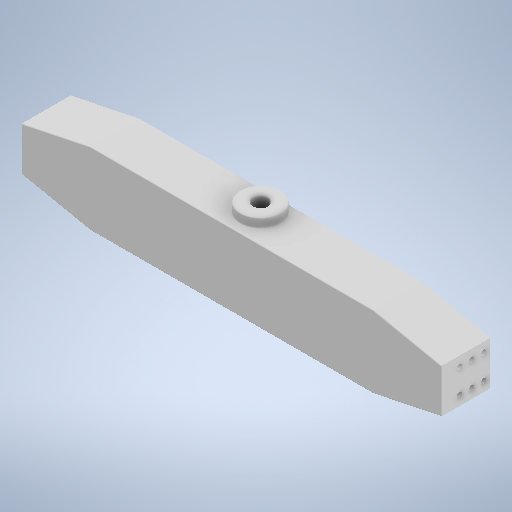
# Autodesk Inventor part: pret_handler_v2
Saved by Autodesk Inventor 2025.2 (Build 292293000, 293)
## iProperties
Created: 2026-04-10
Part Number: pret_handler_v2
Material: Ogólny
Document SubType Name: Modeling
Designer: Admin
Density: 1 g/cm^3
Appearance: Domyślna
Author: Admin
Autodesk Inventor part; units mm, degrees
ref_plane "YZ Plane" through (0, 0, 0) normal (1, 0, 0) x (0, 1, 0)
ref_plane "XZ Plane" through (0, 0, 0) normal (0, 1, 0) x (-1, 0, 0)
ref_plane "XY Plane" through (0, 0, 0) normal (0, 0, 1) x (1, 0, 0)
sketch "Szkic1" plane through (0, 0, 0) normal (0, 0, 1) x (1, 0, 0)
  line L0 (-120, 12.5) -> (-120, -12.5)
  line L1 (-120, 12.5) -> (-80.837, 20.64)
  line L2 (-80.837, 20.64) -> (0, 20.64)
  line L3 (-120, 0) -> (120, 0) construction
  line L4 (-120, -12.5) -> (-80.837, -20.64)
  line L5 (-80.837, -20.64) -> (0, -20.64)
  line L6 (0, 20.64) -> (0, -20.64) construction
  line L7 (120, 12.5) -> (120, -12.5)
  line L8 (120, 12.5) -> (80.837, 20.64)
  line L9 (80.837, 20.64) -> (0, 20.64)
  line L10 (120, -12.5) -> (80.837, -20.64)
  line L11 (80.837, -20.64) -> (0, -20.64)
  point P0 (0, 0)
  point P1 (0, 0)
  dimension "d0" = 25
  dimension "d1" = 40
  dimension "d2" = 80.837
  dimension "d4" = 39.163
  constraints: 24 end point, 6 symmetric about line, 3 midpoint, 2 horizontal, 2 vertical, 1 coincident
  measures "d0" distance of L0.start L0.end
  measures "d1" distance of L0.start L1.end
  measures "d2" distance of L1.end L2.end
  measures "d4" horizontal distance of L0.end L4.end
extrude "Wyciągnięcie proste1" add sketch "Szkic1" along normal blind 28
sketch "Szkic2" plane through (0, 0, 0) normal (0, 0, -1) x (-1, 0, 0)
  line L0 (120, 12.5) -> (120, -12.5) projected
  line L1 (-120, -12.5) -> (-120, 12.5) construction
  line L2 (80.837, -20.64) -> (-80.837, -20.64) construction
  line L3 (120, -12.5) -> (80.837, -20.64) construction
  line L4 (120, 12.5) -> (120, -12.5) construction
  line L5 (80.837, 20.64) -> (120, 12.5) construction
  line L6 (-80.837, 20.64) -> (80.837, 20.64) construction
  line L7 (-120, 12.5) -> (-80.837, 20.64) construction
  line L8 (-80.837, -20.64) -> (-120, -12.5) construction
  line L9 (80.4771, -17.14) -> (-80.4771, -17.14)
  line L10 (-80.4771, -17.14) -> (-116.5, -9.6527)
  line L11 (-116.5, -9.6527) -> (-116.5, 9.6527)
  line L12 (-116.5, 9.6527) -> (-80.4771, 17.14)
  line L13 (-80.4771, 17.14) -> (80.4771, 17.14)
  line L14 (80.4771, 17.14) -> (116.5, 9.6527)
  line L15 (116.5, 9.6527) -> (116.5, -9.6527)
  line L16 (116.5, -9.6527) -> (80.4771, -17.14)
  line L17 (-11.5, 11.5) -> (11.5, 11.5)
  line L18 (11.5, 11.5) -> (11.5, -11.5)
  line L19 (11.5, -11.5) -> (-11.5, -11.5)
  line L20 (-11.5, -11.5) -> (-11.5, 11.5)
  line L21 (-11.5, 11.5) -> (11.5, -11.5) construction
  line L22 (11.5, 11.5) -> (-11.5, -11.5) construction
  line L23 (23, -17.14) -> (23, 17.14)
  line L24 (-23, 17.14) -> (-23, -17.14)
  point P0 (0, 0)
  dimension "d7" = 3.5
  dimension "d8" = 23
  dimension "d9" = 23
  dimension "d10" = 23
  dimension "d11" = 23
  dimension "d12" = 46
  dimension "d13" = 34.28
  constraints: 32 end point, 3 parallel, 2 midpoint, 2 perpendicular, 2 point on line, 1 horizontal, 7 other
  measures "d7" distance between parallel lines of L3 L16
  measures "d8" distance of L18.end L19.end
  measures "d9" distance of L17.end L18.end
  measures "d10" distance from line of point (0, 0) L23
  measures "d11" distance from line of point (0, 0) L24
  measures "d12" distance of L24.end L23.start
  measures "d13" distance of L24.start L24.end
extrude "Wyciągnięcie proste2" cut sketch "Szkic2" against normal blind 22 contours L9 L23 L13 L14 L15 L16 | L9 L10 L11 L12 L13 L24
extrude "Wyciągnięcie proste3" cut sketch "Szkic2" against normal blind 23 contours L17 L18 L19 L20
sketch "Szkic3" plane through (0, 0, 22) normal (0, 0, -1) x (-1, 0, 0)
  line L0 (-116.5, -9.6527) -> (-116.5, 9.6527) projected
  line L1 (-116.5, 0) -> (-114, 0) construction
  line L2 (-80.4771, -17.14) -> (-116.5, -9.6527) projected
  line L3 (-114, -10.1723) -> (-114, 10.1723)
  line L4 (-116.5, 9.6527) -> (-80.4771, 17.14) projected
  line L5 (-116.5, 9.6527) -> (-114, 10.1723)
  line L6 (-116.5, 9.6527) -> (-116.5, -9.6527)
  line L7 (-114, -10.1723) -> (-116.5, -9.6527)
  point P0 (0, 0)
  dimension "d18" = 2.5
  dimension "d19" = 20.3446
  constraints: 10 end point, 3 collinear, 2 point on line, 1 horizontal, 1 midpoint, 1 vertical
  measures "d18" distance of L1.start L1.end
  measures "d19" distance of L3.start L3.end
extrude "Wyciągnięcie proste4" add sketch "Szkic3" along normal blind 22
ref_plane "Płaszczyzna konstrukcyjna1" through (0, -11.5, 0) normal (1, 0, 0) x (0, 0, -1)
mirror "Odbij1" about plane through (0, -11.5, 0) normal (1, 0, 0) of "Wyciągnięcie proste4"
sketch "Szkic4" plane through (-80.837, 20.64, 0) normal (0, 1, 0) x (1, 0, 0)
  line L0 (69.337, 0) -> (69.337, -23) construction
  circle A0 centre (80.837, -11.5) radius 4.25
  line L1 (161.674, 0) -> (0, 0) projected
  line L2 (0, 0) -> (161.674, 0) projected
  circle A1 centre (80.837, -11.5) radius 11.5
  point P0 (80.837, 0)
  dimension "d51" = 8.5
  dimension "d52" = 23
  constraints: 2 centre point, 2 coincident, 1 midpoint, 1 tangent, 1 vertical alignment
  measures "d51" diameter of A0
  measures "d52" diameter of A1
extrude "Wyciągnięcie proste5" add sketch "Szkic4" along normal blind 5
extrude "Wyciągnięcie proste6" cut sketch "Szkic4" against normal through all contours A0
ref_plane "Płaszczyzna konstrukcyjna2" through (-11.5, 0, 0) normal (0, 1, 0) x (1, 0, 0)
mirror "Odbij2" about plane through (-11.5, 0, 0) normal (0, 1, 0) of "Wyciągnięcie proste5"
fillet "Zaokrąglenie1" radius 0.5 12 edges at (23, 0, 0) (51.7386, 17.14, 0) (97.2386, 13.6561, 0) (114, 0, 0) (97.2386, -13.6561, 0) (51.7386, -17.14, 0) (-23, 0, 0) (-51.7386, 17.14, 0) (-97.2386, 13.6561, 0) (-114, 0, 0) (-97.2386, -13.6561, 0) (-51.7386, -17.14, 0)
sketch "Szkic5" plane through (120, -12.5, 0) normal (1, 0, 0) x (0, 0, -1)
  circle A0 centre (-3.75, 19.5) radius 1.5
  line L0 (0, 25) -> (-28, 25) projected
  line L1 (0, 0) -> (0, 25) projected
  circle A1 centre (-10.75, 19.5) radius 1.5
  circle A2 centre (-17.75, 19.5) radius 1.5
  circle A3 centre (-3.75, 5.5) radius 1.5
  circle A4 centre (-10.75, 5.5) radius 1.5
  circle A5 centre (-17.75, 5.5) radius 1.5
  point P0 (0, 12.5)
  dimension "d31" = 3
  dimension "d32" = 5.5
  dimension "d33" = 3.75
  dimension "d36" = 7
  dimension "d39" = 14
  constraints: 6 centre point, 1 horizontal, 1 vertical, 10 other
  measures "d31" diameter of A0
  measures "d32" distance from line of L0 A0.centre
  measures "d33" distance from line of L1 A0.centre
  measures "d36" distance of A0.centre A1.centre
  measures "d39" distance of A0.centre A3.centre
extrude "Wyciągnięcie proste7" cut sketch "Szkic5" against normal blind 6
sketch "Szkic6" plane through (-11.5, 11.5, 0) normal (0, -1, 0) x (1, 0, 0)
  line L0 (0, 23) -> (23, 23) projected
  line L1 (11.5, 0) -> (11.5, 23) construction
  circle A0 centre (11.5, 11.5) radius 11.5 projected
  line L2 (23, 0) -> (23, 23) projected
  line L3 (0, 0) -> (0, 23) projected
  point P0 (0, 11.5)
  point P1 (11.5, 23)
  point P2 (23, 11.5)
  constraints: 2 end point, 1 vertical
extrude "Wyciągnięcie proste8" add sketch "Szkic6" along normal up to surface (23 mm away) contours L0 A0 L3 | L0 L2 A0
sketch "Szkic7" plane through (0, 0, 0) normal (0, 0, -1) x (-1, 0, 0)
  circle A0 centre (-17.5, 15.64) radius 1.5
  line L0 (-22.5, -17.64) -> (-22.5, 17.64) projected
  line L1 (-80.837, 20.64) -> (0, 20.64) projected
  line L2 (-11.5, 11.5) -> (11.5, 11.5) projected
  line L3 (-4.25, -11.5) -> (4.25, -11.5) projected
  line L4 (-11.5, -11.5) -> (-11.5, 11.5) construction
  line L5 (11.5, 11.5) -> (11.5, -11.5) construction
  circle A1 centre (17.5, 15.64) radius 1.5
  circle A2 centre (-17.5, -15.64) radius 1.5
  circle A3 centre (17.5, -15.64) radius 1.5
  point P0 (0, 0)
  dimension "d60" = 3
  dimension "d61" = 5
  dimension "d62" = 5
  dimension "d63" = 35
  dimension "d65" = 31.28
  dimension "d66" = 31.28
  dimension "d67" = 6
  dimension "d68" = 27.14
  dimension "d69" = 6
  constraints: 4 centre point, 3 equal radius
  measures "d60" diameter of A0
  measures "d61" distance from line of A0.centre L0
  measures "d62" distance from line of L1 A0.centre
  measures "d63" distance of A3.centre A2.centre
  measures "d65" distance of A0.centre A2.centre
  measures "d66" distance of A3.centre A1.centre
  measures "d67" distance from line of A1.centre L5
  measures "d68" distance from line of A1.centre L3
  measures "d69" distance from line of A3.centre L5
hole "Otwór2" at (17.5, 15.64, 0) at (-17.5, 15.64, 0) at (17.5, -15.64, 0) at (-17.5, -15.64, 0) direction (0, 0, 1) diameter 3.242 depth 11.8 tip angle 118 counterbore diameter 3.9 counterbore depth 1.8 thread size "M4x0.7" class "6H" standard "ISO Metric profile"
ref_plane "Płaszczyzna konstrukcyjna3" through (0, -11.5, 0) normal (-1, 0, 0) x (0, 0, 1)
ref_plane "Płaszczyzna konstrukcyjna4" through (0, -11.5, 0) normal (-1, 0, 0) x (0, 0, 1)
mirror "Odbij4" about plane through (0, -11.5, 0) normal (-1, 0, 0) of "Wyciągnięcie proste7"
fillet "Zaokrąglenie2" radius 0.5 8 edges at (100.4185, -16.57, 28) (0, -20.64, 28) (-100.4185, -16.57, 28) (-100.4185, 16.57, 28) (0, 20.64, 28) (100.4185, 16.57, 28) (120, 0, 28) (-120, 0, 28)
fillet "Zaokrąglenie3" radius 0.5 3 edges at (-11.5, 25.64, 11.5) (8.1317, 20.64, 3.3683) (-8.1317, 20.64, 19.6317)
fillet "Zaokrąglenie4" radius 0.5 1 edges at (-4.25, 25.64, 11.5)
fillet "Zaokrąglenie5" radius 0.5 4 edges at (-11.5, -25.64, 11.5) (-8.1317, -20.64, 19.6317) (8.1317, -20.64, 3.3683) (-4.25, -25.64, 11.5)
